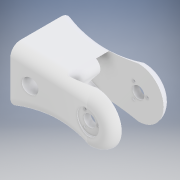
# Autodesk Inventor part: AA010
Saved by Autodesk Inventor 2017 SP1 (Build 210196100, 196)
## iProperties
Created: 2017-09-29
Part Number: AA010
Material: ABS Plastic
Document SubType Name: Modeling
Designer: Zach
Density: 1.06 g/cm^3
Appearance: CR White
Author: Zach
Autodesk Inventor part; units mm, degrees
ref_plane "YZ Plane" through (0, 0, 0) normal (1, 0, 0) x (0, 1, 0)
ref_plane "XZ Plane" through (0, 0, 0) normal (0, 1, 0) x (-1, 0, 0)
ref_plane "XY Plane" through (0, 0, 0) normal (0, 0, 1) x (1, 0, 0)
sketch "Sketch1" plane through (0, 0, 0) normal (0, 0, 1) x (1, 0, 0)
  line L0 (0, 0) -> (0, 105)
  circle A0 centre (32.4, 52.5) radius 2.5
  circle A1 centre (145, 52.5) radius 11.25
  circle A2 centre (145, 52.5) radius 47.5 construction
  arc A3 (145, 5) -> (0, 0) centre (84.2999, -339.6962) ccw
  arc A4 (0, 105) -> (145, 100) centre (84.2999, 444.6962) ccw
  arc A5 (145, 5) -> (145, 100) centre (145, 52.5) ccw
  point P0 (0, 52.5)
  dimension "d0" = 105
  dimension "d1" = 5
  dimension "d2" = 22.5
  dimension "d3" = 112.6
  dimension "d4" = 95
  dimension "d5" = 145
  dimension "d6" = 350
  dimension "d7" = 350
  constraints: 8 point on circle, 6 centre point, 2 end point, 2 horizontal alignment, 2 vertical alignment, 1 coincident, 1 concentric, 1 midpoint, 1 vertical
  measures "d0" distance of L0.start L0.end
  measures "d1" diameter of A0
  measures "d2" diameter of A1
  measures "d3" distance of A1.centre A0.centre
  measures "d4" diameter of A2
  measures "d5" distance of point (0, 52.5) A2.centre
  measures "d6" radius of A3
  measures "d7" radius of A4
extrude "Extrusion1" add sketch "Sketch1" along normal blind 115
sketch "Sketch2" plane through (0, 0, 0) normal (0, 1, 0) x (-1, 0, 0)
  line L0 (0, 0) -> (-145, 0) projected
  arc A0 (0, 0) -> (-145, 0) centre (-72.5, -342.4087) ccw
  line L1 (-145, 115) -> (0, 115) projected
  arc A1 (-145, 115) -> (0, 115) centre (-72.5, 457.4087) ccw
  dimension "d10" = 350
  dimension "d11" = 350
  constraints: 4 point on circle, 2 centre point
  measures "d10" radius of A0
  measures "d11" radius of A1
extrude "Extrusion2" cut sketch "Sketch2" along normal through all
ref_plane "Work Plane1" through (0, 0, 57.5) normal (0, 0, 1) x (1, 0, 0)
sketch "Sketch3" plane through (0, 0, 57.5) normal (0, 0, 1) x (1, 0, 0)
  arc A0 (145, 41.25) -> (145, 63.75) centre (145, 52.5) ccw projected
  arc A1 (145, 41.25) -> (145, 63.75) centre (145, 52.5) ccw projected
  circle A2 centre (145, 52.5) radius 52.5
  point P0 (0, 0)
  dimension "d15" = 105
  constraints: 1 centre point, 1 coincident
  measures "d15" diameter of A2
extrude "Extrusion3" cut sketch "Sketch3" along normal mid plane 79
fillet "Fillet2" radius 15 2 edges at (115.7763, 96.1145, 57.5) (115.7763, 8.8855, 57.5)
fillet "Fillet3" radius 20 4 edges at (71.9844, 94.913, 7.5909) (71.9844, 94.913, 107.4091) (71.9843, 10.087, 107.4091) (71.9843, 10.087, 7.5909)
fillet "Fillet4" radius 20 2 edges at (192.5, 52.5, 115) (192.5, 52.5, 0)
sketch "Sketch4" plane through (0, 19.5779, 115) normal (-1, 0, 0) x (0, 0, 1)
  line L0 (-72, 12.9221) -> (-97, 12.9221)
  line L1 (-97, 12.9221) -> (-97, 52.9221)
  line L2 (-97, 52.9221) -> (-72, 52.9221)
  line L3 (-72, 52.9221) -> (-72, 12.9221)
  line L4 (-95.5772, -19.5779) -> (-19.4228, -19.5779) projected
  line L5 (-115, 0) -> (-115, 65.8443) projected
  line L6 (-97, -14.5765) -> (-97, -7.145) projected
  line L7 (-97, 80.4208) -> (-97, -14.5765) projected
  line L8 (-97, 72.9893) -> (-97, 80.4208) projected
  line L9 (-97, 54.076) -> (-97, 72.9893) projected
  line L10 (-97, 11.7683) -> (-97, 54.076) projected
  line L11 (-97, -7.145) -> (-97, 11.7683) projected
  line L12 (-97, 21.6721) -> (-97, 44.1721) projected
  line L13 (-18, 44.1721) -> (-18, 21.6721) projected
  line L14 (-18, -7.145) -> (-18, -14.5765) projected
  line L15 (-18, 11.7683) -> (-18, -7.145) projected
  line L16 (-18, 54.076) -> (-18, 11.7683) projected
  line L17 (-18, 72.9893) -> (-18, 54.076) projected
  line L18 (-18, 80.4208) -> (-18, 72.9893) projected
  line L19 (-18, -14.5765) -> (-18, 80.4208) projected
  point P0 (-115, -19.5779)
  point P1 (-84.5, 12.9221)
  point P2 (-57.5, -19.5779)
  point P3 (-97, 32.9221)
  point P4 (-115, 32.9221)
  dimension "d21" = 25
  dimension "d22" = 40
  constraints: 8 end point, 5 midpoint, 2 parallel, 1 horizontal, 1 horizontal alignment, 1 perpendicular
  measures "d21" distance of L1.end L2.end
  measures "d22" distance of L0.end L1.end
extrude "Extrusion4" cut sketch "Sketch4" against normal through all
sketch "Sketch5" plane through (0, 19.5779, 115) normal (-1, 0, 0) x (0, 0, 1)
  circle A0 centre (-57.5, 32.9221) radius 38.5
  line L0 (-95.5772, -19.5779) -> (-19.4228, -19.5779) projected
  line L1 (-115, 0) -> (-115, 65.8443) projected
  point P0 (-115, -19.5779)
  point P1 (-57.5, -19.5779)
  point P2 (-115, 32.9221)
  dimension "d25" = 77
  constraints: 2 midpoint, 1 centre point, 1 horizontal alignment, 1 vertical alignment
  measures "d25" diameter of A0
extrude "Extrusion5" cut sketch "Sketch5" against normal blind 17.5
sketch "Sketch6" plane through (0, 0, 0) normal (0, 0, -1) x (-1, 0, 0)
  circle A0 centre (-145, 52.5) radius 22.5
  arc A1 (-145, 63.75) -> (-145, 41.25) centre (-145, 52.5) ccw projected
  point P0 (0, 0)
  dimension "d28" = 45
  constraints: 1 centre point, 1 concentric
  measures "d28" diameter of A0
extrude "Extrusion6" cut sketch "Sketch6" against normal blind 5
sketch "Sketch7" plane through (0, 0, 115) normal (0, 0, 1) x (1, 0, 0)
  circle A0 centre (145, 52.5) radius 22.5
  arc A1 (145, 41.25) -> (145, 63.75) centre (145, 52.5) ccw projected
  point P0 (0, 0)
  dimension "d31" = 45
  constraints: 1 centre point, 1 concentric
  measures "d31" diameter of A0
extrude "Extrusion7" cut sketch "Sketch7" against normal blind 5
sketch "Sketch8" plane through (145, 52.5, 110) normal (0, 0, 1) x (1, 0, 0)
  circle A0 centre (17, 0) radius 2.5
  circle A1 centre (0, 0) radius 11.25 construction
  circle A2 centre (-8.5, 14.7224) radius 2.5
  circle A3 centre (-8.5, -14.7224) radius 2.5
  point P0 (-145, -52.5)
  dimension "d34" = 5
  dimension "d35" = 17
  dimension "d38" = 360
  constraints: 3 centre point, 1 horizontal alignment, 7 other
  measures "d34" diameter of A0
  measures "d35" distance of A0.centre A1.centre
extrude "Extrusion8" cut sketch "Sketch8" against normal through all
sketch "Sketch9" plane through (0, 19.5779, 115) normal (-1, 0, 0) x (0, 0, 1)
  arc A0 (-90.3976, 12.9221) -> (-90.3976, 52.9221) centre (-57.5, 32.9221) ccw construction
  circle A1 centre (-57.5, 32.9221) radius 12.5
  circle A2 centre (-35.8494, 20.4221) radius 2.5
  circle A3 centre (-35.8494, 45.4221) radius 2.5
  circle A4 centre (-57.5, 57.9221) radius 2.5
  circle A5 centre (-79.1506, 45.4221) radius 2.5
  circle A6 centre (-79.1506, 20.4221) radius 2.5
  circle A7 centre (-57.5, 7.9221) radius 2.5
  point P0 (-115, -19.5779)
  dimension "d42" = 25
  dimension "d43" = 5
  dimension "d44" = 25
  dimension "d47" = 360
  constraints: 7 centre point, 1 coincident, 1 vertical alignment, 13 other
  measures "d42" diameter of A1
  measures "d43" diameter of A2
  measures "d44" distance of A0.centre A2.centre
extrude "Extrusion9" cut sketch "Sketch9" against normal blind 25 contours A2 | A3 | A4 | A7
sketch "Sketch10" plane through (17.5, 19.5779, 115) normal (-1, 0, 0) x (0, 0, 1)
  arc A0 (-90.3976, 12.9221) -> (-90.3976, 52.9221) centre (-57.5, 32.9221) ccw projected
  circle A1 centre (-57.5, 32.9221) radius 12.5
  point P0 (-115, -19.5779)
  dimension "d51" = 25
  constraints: 1 centre point, 1 coincident
  measures "d51" diameter of A1
extrude "Extrusion10" cut sketch "Sketch10" against normal through all
sketch "Sketch11" plane through (17.5, 19.5779, 115) normal (-1, 0, 0) x (0, 0, 1)
  circle A0 centre (-57.5, 32.9221) radius 12.5 construction
  line L0 (-72, 12.9221) -> (-72, 52.9221) projected
  line L1 (-90.3976, 12.9221) -> (-72, 12.9221) projected
  line L2 (-72, 52.9221) -> (-90.3976, 52.9221) projected
  line L3 (-72, 52.9221) -> (-52.4837, 44.3714)
  line L4 (-72, 52.9221) -> (-72, 12.9221) projected
  line L5 (-72, 12.9221) -> (-52.4837, 21.4728)
  arc A1 (-52.4837, 21.4728) -> (-52.4837, 44.3714) centre (-57.5, 32.9221) ccw
  point P0 (-115, -19.5779)
  constraints: 4 end point, 4 point on circle, 4 tangent, 1 centre point
extrude "Extrusion11" cut sketch "Sketch11" against normal through all
sketch "Sketch12" plane through (0, 0, 18) normal (0, 0, 1) x (1, 0, 0)
  circle A0 centre (32.4, 52.5) radius 2.5 projected
  line L0 (17.5, 72.5) -> (0, 72.5) projected
  line L1 (0, 32.5) -> (17.5, 32.5) projected
  circle A1 centre (32.4, 52.5) radius 14.9 construction
  circle A2 centre (32.4, 52.5) radius 10 construction
  line L2 (17.5, 32.5) -> (17.5, 72.5) construction
  line L3 (32.4, 62.5) -> (32.4, 67.4)
  line L4 (32.4, 42.5) -> (32.4, 37.6)
  arc A3 (32.4, 67.4) -> (32.4, 37.6) centre (32.4, 52.5) ccw
  arc A4 (32.4, 62.5) -> (32.4, 42.5) centre (32.4, 52.5) ccw
  point P0 (0, 0)
  point P1 (17.5, 52.5)
  dimension "d71" = 20
  constraints: 10 point on circle, 6 end point, 4 centre point, 2 coincident, 2 point on line, 2 vertical, 1 concentric, 1 midpoint, 1 vertical alignment, 2 other
  measures "d71" diameter of A2
extrude "Extrusion12" add sketch "Sketch12" along normal blind 25 contours A4 L4 A3 L3
sketch "Sketch14" plane through (0, 0, 43) normal (0, 0, 1) x (1, 0, 0)
  circle A0 centre (32.4, 52.5) radius 2.5 projected
  circle A1 centre (32.4, 52.5) radius 14.9
  arc A2 (32.4, 67.4) -> (32.4, 37.6) centre (32.4, 52.5) ccw projected
  line L0 (23.9, 52.5) -> (40.9, 52.5) construction
  circle A3 centre (23.9, 52.5) radius 1.5
  circle A4 centre (40.9, 52.5) radius 1.5
  point P0 (0, 0)
  dimension "d73" = 17
  dimension "d74" = 3
  dimension "d75" = 3
  constraints: 4 coincident, 2 centre point, 2 end point, 1 horizontal, 1 midpoint, 1 vertical alignment, 2 other
  measures "d73" distance of L0.start L0.end
  measures "d74" diameter of A3
  measures "d75" diameter of A4
extrude "Extrusion13" add sketch "Sketch14" along normal blind 5
sketch "Sketch15" plane through (32.4, 52.5, 48) normal (0, 0, 1) x (1, 0, 0)
  circle A0 centre (0, 0) radius 2.5 projected
  circle A1 centre (0, 0) radius 14
  dimension "d81" = 28
  constraints: 1 centre point, 1 coincident
  measures "d81" diameter of A1
extrude "Extrusion14" cut sketch "Sketch15" along normal through all
sketch "Sketch16" plane through (32.4, 52.5, 48) normal (0, 0, 1) x (1, 0, 0)
  circle A0 centre (0, 0) radius 2.5 projected
  circle A1 centre (0, 0) radius 4
  point P0 (-32.4, -52.5)
  dimension "d76" = 8
  constraints: 1 centre point, 1 coincident
  measures "d76" diameter of A1
extrude "Extrusion15" cut sketch "Sketch16" against normal blind 3
sketch "Sketch17" plane through (32.4, 52.5, 48) normal (0, 0, 1) x (1, 0, 0)
  circle A0 centre (-8.5, 0) radius 1.5 projected
  circle A1 centre (8.5, 0) radius 1.5 projected
  point P0 (-32.4, -52.5)
  point P1 (-10, 0)
  constraints: 1 horizontal alignment
extrude "Extrusion16" cut sketch "Sketch17" against normal through all
sketch "Sketch18" plane through (0, 0, 43) normal (0, 0, -1) x (-1, 0, 0)
  line L0 (-32.4, 37.6) -> (-32.4, 42.5) projected
  arc A0 (-32.4, 42.5) -> (-22.4, 52.5) centre (-32.4, 52.5) ccw projected
  circle A1 centre (-23.9, 52.5) radius 1.5 projected
  arc A2 (-22.4, 52.5) -> (-32.4, 62.5) centre (-32.4, 52.5) ccw projected
  line L1 (-32.4, 62.5) -> (-32.4, 67.4) projected
  arc A3 (-32.4, 67.4) -> (-32.4, 37.6) centre (-32.4, 52.5) ccw projected
  circle A4 centre (-40.9, 52.5) radius 1.5 projected
  circle A5 centre (-32.4, 52.5) radius 2.5 projected
  circle A6 centre (-32.4, 52.5) radius 13
  point P0 (0, 0)
  dimension "d82" = 26
  constraints: 1 centre point, 1 coincident, 1 horizontal alignment
  measures "d82" diameter of A6
extrude "Extrusion17" cut sketch "Sketch18" along normal through all contours A6 L1 A2 A0 L0 | L0 A0 A2 L1 A6
sketch "Sketch19" plane through (0, 19.5779, 115) normal (-1, 0, 0) x (0, 0, 1)
  arc A0 (-90.3976, 12.9221) -> (-90.3976, 52.9221) centre (-57.5, 32.9221) ccw construction
  line L0 (-97, 52.9221) -> (-90.3976, 52.9221) projected
  line L1 (-97, 12.9221) -> (-97, 52.9221) projected
  line L2 (-90.3976, 12.9221) -> (-97, 12.9221) projected
  arc A1 (-90.3976, 52.9221) -> (-90.3976, 12.9221) centre (-57.5, 32.9221) ccw
  point P0 (-115, -19.5779)
  constraints: 2 point on circle, 1 centre point, 1 coincident
extrude "Extrusion18" add sketch "Sketch19" against normal blind 17.5
sketch "Sketch22" plane through (0, 0, 18) normal (0, 0, 1) x (1, 0, 0)
  arc A0 (32.4, 39.5) -> (32.4, 65.5) centre (32.4, 52.5) ccw construction
  circle A1 centre (145, 52.5) radius 11.25 construction
  circle A2 centre (32.4, 52.5) radius 12.5 construction
  circle A3 centre (145, 52.5) radius 60 construction
  line L0 (27.1269, 63.8333) -> (119.6892, 106.9)
  line L1 (27.1269, 41.1667) -> (119.6892, -1.9)
  arc A4 (119.6892, -1.9) -> (119.6892, 106.9) centre (145, 52.5) ccw
  arc A5 (27.1269, 63.8333) -> (27.1269, 41.1667) centre (32.4, 52.5) ccw
  point P0 (0, 0)
  dimension "d92" = 25
  dimension "d93" = 120
  constraints: 8 point on circle, 7 tangent, 4 centre point, 4 end point, 2 coincident
  measures "d92" diameter of A2
  measures "d93" diameter of A3
extrude "Extrusion21" cut sketch "Sketch22" along normal blind 25
sketch "Sketch23" plane through (0, 0, 18) normal (0, 0, 1) x (1, 0, 0)
  circle A0 centre (32.4, 52.5) radius 14.9 construction
  circle A1 centre (136.5, 67.2224) radius 2.5 construction
  circle A2 centre (162, 52.5) radius 2.5 construction
  circle A3 centre (136.5, 37.7776) radius 2.5 construction
  circle A4 centre (145, 52.5) radius 11.25 construction
  line L0 (17.5, 72.5) -> (45.754, 72.5) construction
  line L1 (17.5, 72.5) -> (17.5, 52.5) construction
  arc A5 (32.4, 67.4) -> (17.5, 52.5) centre (32.4, 52.5) ccw construction
  line L2 (32.4, 67.4) -> (32.4, 66.2868) construction
  line L3 (30.3644, 65.3396) -> (32.4, 66.2868) construction
  arc A6 (30.3644, 39.6604) -> (30.3644, 65.3396) centre (32.4, 52.5) ccw construction
  line L4 (32.4, 38.7132) -> (30.3644, 39.6604) construction
  line L5 (32.4, 38.7132) -> (32.4, 37.6) construction
  arc A7 (17.5, 52.5) -> (32.4, 37.6) centre (32.4, 52.5) ccw construction
  line L6 (17.5, 52.5) -> (17.5, 32.5) construction
  line L7 (17.5, 32.5) -> (45.754, 32.5) construction
  line L8 (88.6807, 12.5274) -> (45.754, 32.5) construction
  arc A8 (145.3586, 5.0014) -> (145.3586, 99.9986) centre (145, 52.5) ccw construction
  line L9 (45.754, 72.5) -> (88.6807, 92.4726) construction
  line L10 (30.3644, 65.3396) -> (32.4, 66.2868)
  line L11 (32.4, 72.5) -> (17.5, 72.5)
  line L12 (17.5, 72.5) -> (17.5, 32.5)
  line L13 (30.3644, 39.6604) -> (32.4, 38.7132)
  line L14 (32.4, 32.5) -> (17.5, 32.5)
  arc A9 (30.3644, 65.3396) -> (30.3644, 39.6604) centre (32.4, 52.5) ccw
  line L15 (32.4, 66.2868) -> (45.754, 72.5)
  line L16 (32.4, 38.7132) -> (45.754, 32.5)
  line L17 (32.4, 32.5) -> (45.754, 32.5)
  line L18 (45.754, 72.5) -> (32.4, 72.5)
  point P0 (0, 0)
  point P1 (17.5, 72.5)
  point P2 (17.5, 32.5)
  constraints: 18 end point, 5 collinear, 2 point on circle, 2 point on line, 1 centre point, 1 concentric, 1 perpendicular, 4 other
extrude "Extrusion22" add sketch "Sketch23" along normal blind 30
sketch "Sketch24" plane through (0, 0, 43) normal (0, 0, -1) x (-1, 0, 0)
  circle A0 centre (-40.9, 52.5) radius 1.5 projected
  circle A1 centre (-23.9, 52.5) radius 1.5 projected
  circle A2 centre (-40.9, 52.5) radius 4.5
  circle A3 centre (-23.9, 52.5) radius 4.5
  point P0 (0, 0)
  dimension "d98" = 9
  dimension "d99" = 9
  constraints: 2 centre point, 2 coincident
  measures "d98" diameter of A2
  measures "d99" diameter of A3
extrude "Extrusion23" cut sketch "Sketch24" against normal blind 3
sketch "Sketch21" plane through (0, 0, 57.5) normal (0, 0, 1) x (1, 0, 0)
  line L0 (0, 0) -> (180, 0) construction
  line L1 (180, 0) -> (180, 105) construction
  line L2 (180, 105) -> (0, 105) construction
  line L3 (0, 105) -> (0, 0) construction
  line L4 (180, 105) -> (192.5, 105)
  line L5 (192.5, 105) -> (192.5, 0)
  line L6 (192.5, 0) -> (180, 0)
  line L7 (180, 0) -> (180, 105)
  arc A0 (145.3586, 5.0014) -> (145.3586, 99.9986) centre (145, 52.5) ccw projected
  point P0 (192.5, 52.5)
  dimension "d89" = 180
  constraints: 16 end point, 4 parallel, 2 horizontal, 2 perpendicular, 1 horizontal alignment, 1 midpoint, 1 point on circle
  measures "d89" distance of L2.end L1.end
extrude "Extrusion20" [suppressed]
body "Solid1"
